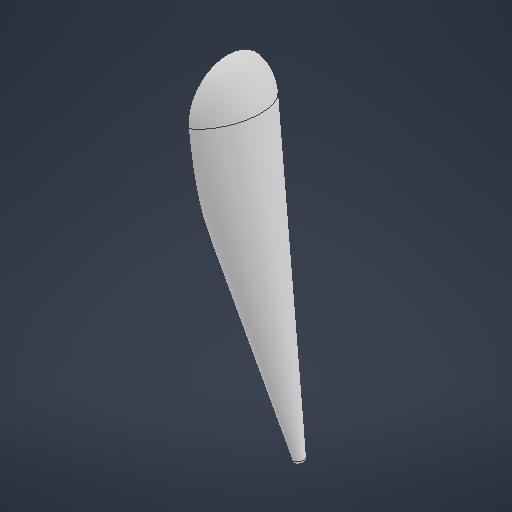
# Autodesk Inventor part: Arm
Saved by Autodesk Inventor 2025.2 (Build 292293000, 293)
## iProperties
Created: 2025-03-31
Part Number: Arm
Material: Generic
Document SubType Name: Modeling
Designer: mylap
Density: 1 g/cm^3
Appearance: Default
Author: mylap
## iProperties of the stored document Arm_3DPrint.ipt
Created: 2025-03-31
Part Number: Arm_3DPrint
Material: Generic
Document SubType Name: Modeling
Designer: mylap
Density: 1 g/cm^3
Appearance: Default
Author: mylap
Autodesk Inventor part; units mm, degrees
ref_plane "YZ Plane" through (0, 0, 0) normal (1, 0, 0) x (0, 1, 0)
ref_plane "XZ Plane" through (0, 0, 0) normal (0, 1, 0) x (-1, 0, 0)
ref_plane "XY Plane" through (0, 0, 0) normal (0, 0, 1) x (1, 0, 0)
sketch "Sketch1" plane through (0, 0, 0) normal (0, 0, 1) x (1, 0, 0)
  line L0 (4.644423, 87.11898) -> (49.09442, 87.11898) construction
  line L1 (49.09442, 87.11898) -> (49.09442, 4.568979) construction
  line L2 (49.09442, 4.568979) -> (4.644423, 4.568979) construction
  line L3 (4.644423, 4.568979) -> (4.644423, 87.11898) construction
  arc A0 (42.010595, 57.266391) -> (39.319274, 61.030194) centre (38.708835, 57.749576) ccw
  line L4 (42.010595, 58.232761) -> (45.522994, 35.63788)
  line L5 (45.383124, 35.370458) -> (45.05229, 35.209512)
  line L6 (44.703976, 35.347068) -> (39.602571, 48.666303)
  line L7 (39.602571, 48.666303) -> (39.319274, 61.030194)
  arc A1 (44.703976, 35.347068) -> (45.05229, 35.209512) centre (44.941174, 35.437917) ccw
  arc A2 (45.383124, 35.370458) -> (45.522994, 35.63788) centre (45.272008, 35.598864) ccw
  line L8 (45.217707, 35.289985) -> (38.708835, 57.749576)
  circle A3 centre (38.708835, 57.749576) radius 3.336928
  line L9 (38.708835, 57.749576) -> (37.78, 60.954627)
  point P0 (0, 0)
  point P1 (39.453305, 55.180701)
  point P2 (39.637671, 54.544525)
  point P3 (39.468894, 54.500361)
  dimension "d1" = 0.254
  constraints: 12 end point, 7 point on circle, 4 tangent, 3 centre point, 1 coincident, 1 equal radius, 1 midpoint, 6 other
  measures "d1" radius of A1
sketch "Sketch1 outline for Revolution1" plane through (0, 0, 0) normal (0, 0, 1) x (1, 0, 0)
  arc A0 (45.383124, 35.370458) -> (45.522994, 35.63788) centre (45.272008, 35.598864) ccw
  line L0 (45.217707, 35.289985) -> (45.383124, 35.370458)
  line L1 (38.708835, 57.749576) -> (45.217707, 35.289985)
  line L2 (37.78, 60.954627) -> (38.708835, 57.749576)
  arc A1 (39.319274, 61.030194) -> (37.78, 60.954627) centre (38.708835, 57.749576) ccw
  arc A2 (42.010595, 58.232761) -> (39.319274, 61.030194) centre (38.708835, 57.749576) ccw
  line L3 (45.522994, 35.63788) -> (42.010595, 58.232761)
revolve "Revolution1" add sketch "Sketch1 outline for Revolution1" angle 360 about axis through (45.217707, 35.289985, 0) along (-0.2783505, 0.9604796, 0)
extrude "Extrusion1" cut sketch "Sketch1" along normal mid plane 25.4 contours A3 L8 L7 A0 | A0 L4 A2 L5 L8 A3 | A3 L7 L8 | L8 L5 A1 L6 L7 A3 keep common part
sketch "Sketch2" plane through (0, 0, 0) normal (0, 0, 1) x (1, 0, 0)
  circle A0 centre (39.000074, 58.328695) radius 1.27
  line L0 (39.319274, 61.030194) -> (39.400703, 57.476405)
  line L1 (37.730074, 58.328695) -> (40.270074, 58.328695)
  point P0 (0, 0)
  point P1 (39.381174, 58.328695)
  point P2 (39.353222, 59.548608)
  dimension "d6" = 2.54
  dimension "d7" = 0.381
  constraints: 2 end point, 2 point on circle, 1 centre point, 1 horizontal
  measures "d6" diameter of A0
  measures "d7" distance from line of L0 A0.centre
revolve "Revolution2" add sketch "Sketch2" angle 360 about axis through (37.730074, 58.328695, 0) along (1, 0, 0) contours L1 A0
body "Solid1"
